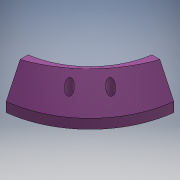
# Autodesk Inventor part: connectro_best
Saved by Autodesk Inventor 2017 (Build 210142000, 142)
## iProperties
Created: 2017-05-24
Part Number: connectro_best
Material: Ogólny
Document SubType Name: Modeling
Designer: Speed King
Density: 1 g/cm^3
Appearance: Gładki - fioletowy
Author: Speed King
Autodesk Inventor part; units mm, degrees
ref_plane "YZ Plane" through (0, 0, 0) normal (1, 0, 0) x (0, 1, 0)
ref_plane "Płaszczyzna konstrukcyjna1" through (0, 0, 0) normal (0, 0, 1) x (1, 0, 0)
sketch "Szkic1" plane through (0, 0, 0) normal (0, 0, 1) x (1, 0, 0)
  arc A0 (15, -100.85) -> (100.85, -15) centre (0, 0) ccw projected
  arc A1 (15, -131.0443) -> (131.0443, -15) centre (0, 0) ccw projected
  line L0 (100.85, -15) -> (111.85, -15) projected
  line L1 (15, -100.85) -> (15, -111.85) projected
  line L2 (15.2, -100.8201) -> (15.2, -131.0213)
  line L3 (100.8201, -15.2) -> (131.0213, -15.2)
  point P0 (0, 0)
  dimension "d0" = 0.2
  dimension "d1" = 0.2
  constraints: 4 end point, 4 point on circle, 2 parallel
  measures "d0" distance between parallel lines of L2 L1
  measures "d1" distance between parallel lines of L3 L0
extrude "Wyciągnięcie proste1" add sketch "Szkic1" along normal up to surface (13.2464 mm away)
sketch "Szkic2" plane through (100.8201, -15.2, 13.2464) normal (0, 0, 1) x (1, 0, 0)
  line L0 (0, 0) -> (30.2012, 0) projected
  arc A0 (-85.6201, -85.6201) -> (0, 0) centre (-100.8201, 15.2) ccw projected
  line L1 (-85.6201, -115.8213) -> (-85.6201, -85.6201) projected
  arc A1 (-85.6201, -115.8213) -> (30.2012, 0) centre (-100.8201, 15.2) ccw projected
ref_plane "Płaszczyzna konstrukcyjna2" through (15, -111.85, 54) normal (0, 0, 1) x (1, 0, 0)
sketch "Szkic3" plane through (15, -111.85, 54) normal (0, 0, 1) x (1, 0, 0)
  arc A0 (0.2, 11.0299) -> (85.8201, 96.65) centre (-15, 111.85) ccw projected
  line L0 (0.2, -19.1713) -> (0.2, 11.0299) projected
  line L1 (85.8201, 96.65) -> (116.0213, 96.65) projected
  line L2 (0.2, 11.0299) -> (0.2, 0.0299)
  line L3 (0.2, -19.1713) -> (0.2, 11.0299) projected
  line L4 (85.8201, 96.65) -> (116.0213, 96.65) projected
  line L5 (85.8201, 96.65) -> (96.8201, 96.65)
  arc A1 (0.2, 0.0299) -> (96.8201, 96.65) centre (-49.8701, 146.7201) ccw
  point P0 (-15, 111.85)
  dimension "d4" = 11
  dimension "d5" = 11
  dimension "d6" = 155
  constraints: 4 end point, 2 point on circle, 2 point on line, 1 centre point
  measures "d4" distance of L0.end L2.end
  measures "d5" distance of L1.start L5.end
  measures "d6" radius of A1
loft "Wyciągnięcie złożone1" add profiles "Szkic2", "Szkic3"
sketch "Szkic7" plane through (0, 0, 0) normal (0, 0, -1) x (-1, 0, 0)
  line L0 (-109.9472, -18) -> (-109.9472, -15) projected
  line L1 (-108.4654, -20.2226) -> (-109.9472, -18) projected
  line L2 (-115.9472, -15) -> (-115.9472, -18) projected
  line L3 (-115.9472, -18) -> (-117.4289, -20.2226) projected
  arc A0 (-117.4289, -20.2226) -> (-117.0129, -21) centre (-117.0129, -20.5) ccw projected
  line L4 (-117.0129, -21) -> (-108.8814, -21) projected
  arc A1 (-108.8814, -21) -> (-108.4654, -20.2226) centre (-108.8814, -20.5) ccw projected
  line L5 (-100.8201, -15.2) -> (-131.0213, -15.2) projected
  line L6 (-18, -115.9472) -> (-15, -115.9472) projected
  line L7 (-20.2226, -117.4289) -> (-18, -115.9472) projected
  arc A2 (-21, -117.0129) -> (-20.2226, -117.4289) centre (-20.5, -117.0129) ccw projected
  line L8 (-21, -108.8814) -> (-21, -117.0129) projected
  arc A3 (-20.2226, -108.4654) -> (-21, -108.8814) centre (-20.5, -108.8814) ccw projected
  line L9 (-18, -109.9472) -> (-20.2226, -108.4654) projected
  line L10 (-15, -109.9472) -> (-18, -109.9472) projected
  line L11 (-15.2, -131.0213) -> (-15.2, -100.8201) projected
  line L12 (-15, -116.1472) -> (-17.9394, -116.1472)
  line L13 (-17.9394, -116.1472) -> (-20.1117, -117.5953)
  arc A4 (-21.2, -117.0129) -> (-20.1117, -117.5953) centre (-20.5, -117.0129) ccw
  line L14 (-21.2, -117.0129) -> (-21.2, -108.8814)
  arc A5 (-20.1117, -108.299) -> (-21.2, -108.8814) centre (-20.5, -108.8814) ccw
  line L15 (-20.1117, -108.299) -> (-17.9394, -109.7472)
  line L16 (-17.9394, -109.7472) -> (-15, -109.7472)
  line L17 (-109.7472, -15) -> (-109.7472, -17.9394)
  line L18 (-109.7472, -17.9394) -> (-108.299, -20.1117)
  arc A6 (-108.8814, -21.2) -> (-108.299, -20.1117) centre (-108.8814, -20.5) ccw
  line L19 (-108.8814, -21.2) -> (-117.0129, -21.2)
  arc A7 (-117.5953, -20.1117) -> (-117.0129, -21.2) centre (-117.0129, -20.5) ccw
  line L20 (-117.5953, -20.1117) -> (-116.1472, -17.9394)
  line L21 (-116.1472, -17.9394) -> (-116.1472, -15)
  line L22 (-116.1472, -15) -> (-109.7472, -15)
  line L23 (-15, -116.1472) -> (-15, -109.7472)
  point P0 (0, 0)
  dimension "d40" = 0.2
  dimension "d41" = 0.2
  dimension "d42" = 0.2
  constraints: 24 end point, 8 point on circle, 4 centre point, 1 horizontal, 1 perpendicular, 12 other
  measures "d40" distance between parallel lines of L7 L13
  measures "d41" distance between parallel lines of L3 L20
  measures "d42" distance between parallel lines of L18 L1
extrude "Wyciągnięcie proste6" cut sketch "Szkic7" against normal blind 31
sketch "Szkic5" plane through (0, 0, 0) normal (0, 0, -1) x (-1, 0, 0)
  circle A0 centre (-95.0216, -66.5349) radius 2.25 projected
  circle A1 centre (-66.5349, -95.0216) radius 2.25 projected
  point P0 (0, 0)
extrude "Wyciągnięcie proste4" cut sketch "Szkic5" against normal through all
ref_plane "Płaszczyzna konstrukcyjna3" through (0, 0, 12) normal (0, 0, -1) x (-1, 0, 0)
sketch "Szkic6" plane through (0, 0, 12) normal (0, 0, -1) x (-1, 0, 0)
  spline S0 degree 2 poles (-64.2849, -95.0216) (-64.2849, -91.1245) (-67.6599, -93.0731) (-71.0349, -95.0216) (-67.6599, -96.9702) (-64.2849, -98.9188) (-64.2849, -95.0216) knots 0 0 0 0.333333 0.333333 0.666667 0.666667 1 1 1 weights 1 0.5 1 0.5 1 0.5 1 projected
  spline S1 degree 2 poles (-92.7716, -66.5349) (-92.7716, -62.6378) (-96.1466, -64.5863) (-99.5216, -66.5349) (-96.1466, -68.4834) (-92.7716, -70.432) (-92.7716, -66.5349) knots 0 0 0 0.333333 0.333333 0.666667 0.666667 1 1 1 weights 1 0.5 1 0.5 1 0.5 1 projected
  circle A0 centre (-95.0216, -66.5349) radius 2.25 projected
  circle A1 centre (-95.0216, -66.5349) radius 5
  circle A2 centre (-66.5349, -95.0216) radius 2.25 projected
  circle A3 centre (-66.5349, -95.0216) radius 5
  point P0 (0, 0)
  dimension "d22" = 10
  dimension "d23" = 10
  constraints: 2 centre point, 2 coincident, 4 other
  measures "d22" diameter of A1
  measures "d23" diameter of A3
extrude "Wyciągnięcie proste5" cut sketch "Szkic6" against normal through all contours S0 | S1 | A1 | A3
equation "\"d1\" = d0"
